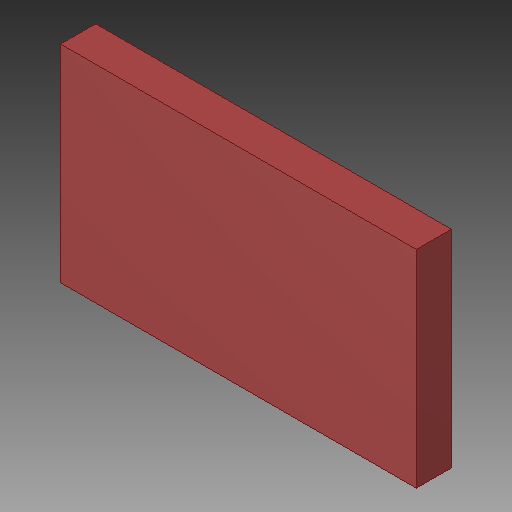
# Autodesk Inventor part: LIDAR
Saved by Autodesk Inventor 2017 (Build 210142000, 142)
## iProperties
Created: 2019-06-13
Part Number: LIDAR
Material: Generic
Document SubType Name: Modeling
Designer: Marc
Density: 1 g/cm^3
Appearance: 6410-04, LIDAR
Author: Marc
Autodesk Inventor part; units mm, degrees
ref_plane "YZ Plane" through (0, 0, 0) normal (1, 0, 0) x (0, 1, 0)
ref_plane "XZ Plane" through (0, 0, 0) normal (0, 1, 0) x (-1, 0, 0)
ref_plane "XY Plane" through (0, 0, 0) normal (0, 0, 1) x (1, 0, 0)
sketch "6410-04, LIDAR_34" plane through (0, 0, 0) normal (0, 0, 1) x (1, 0, 0)
  line L0 (-5.08, 2.9845) -> (5.08, 2.9845)
  line L1 (5.08, 2.9845) -> (5.08, -2.921)
  line L2 (5.08, -2.921) -> (-5.08, -2.921)
  line L3 (-5.08, -2.921) -> (-5.08, 2.9845)
  constraints: 8 end point
extrude "Extrusion1" add sketch "6410-04, LIDAR_34" along normal blind 1
body "Solid1"
